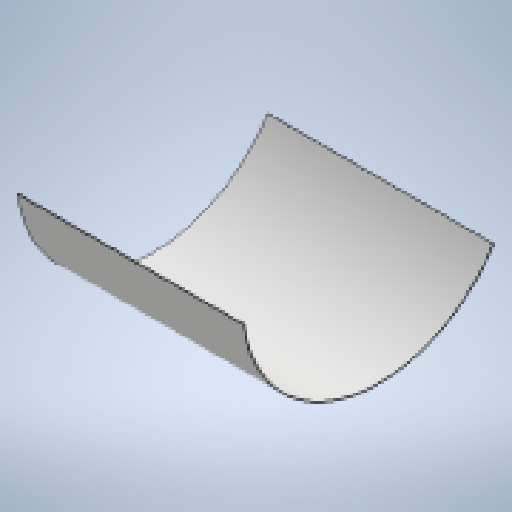
# Autodesk Inventor part: TRM 027 tromel
Saved by Autodesk Inventor 2025 (Build 290162010, 162A)
## iProperties
Created: 2024-08-07
Part Number: TRM 027 tromel
Material: AISI 304
Document SubType Name: Sheet Metal
Designer: admin
Stock Number: ТРМ 017 лист внутри
Density: 8.02768 g/cm^3
Flat Pattern Width: 50 cm
Flat Pattern Length: 73.7116 cm
Flat Pattern Area: 3685.58 cm^2
Sheet Metal Rule: AISI304 2mm Die16
Sheet Metal Width: 500,000 mm
Sheet Metal Length: 737,116 mm
Sheet Metal Area: 368558,013 mm^2
Appearance: Default
d73_joint_angle: 7,40 deg
Author: pokla
Autodesk Inventor part; units mm, degrees
ref_plane "YZ Plane" through (0, 0, 0) normal (1, 0, 0) x (0, 1, 0)
ref_plane "XZ Plane" through (0, 0, 0) normal (0, 1, 0) x (-1, 0, 0)
ref_plane "XY Plane" through (0, 0, 0) normal (0, 0, 1) x (1, 0, 0)
sketch "Sketch7" plane through (0, 0, 0) normal (1, 0, 0) x (0, 1, 0)
  line L0 (297.5, 0) -> (-297.5, 0) construction
  arc A0 (-297.5, 0) -> (253.7716, -121.3509) centre (0, 38.6491) ccw
  line L1 (-253.7716, -121.3509) -> (253.7716, -121.3509) construction
  arc A1 (253.7716, -121.3509) -> (297.5, 0) centre (0, 38.6491) ccw construction
  line L2 (-297.5, 0) -> (-263.5472, -261.3509) construction
  line L3 (-297.5, 0) -> (-297.5, -261.3509) construction
  line L4 (-297.5, -261.3509) -> (165.5032, -261.3509) construction
  line L5 (253.7716, -121.3509) -> (165.5032, -261.3509) construction
  line L6 (-297.5, 0) -> (-310.383, 99.1667)
  line L7 (253.7716, -121.3509) -> (253.7716, 0) construction
  point P0 (0, 0)
  point P1 (0, 0)
  point P2 (-123.3439, -261.3509)
  dimension "d54" = 300
  dimension "d66" = 121.3509
  dimension "d68" = 7.402
  dimension "d69" = 595
  dimension "d70" = 140
  dimension "d72" = 100
  dimension "d73_joint_angle" = 7.402
  dimension "d74" = 147.769
  measures "d54" radius of A0
  measures "d66" distance between parallel lines of L1 L0
  measures "d68" angle of L2 L3
  measures "d69" distance of L0.start L0.end
  measures "d70" distance from line of point (-123.344, -261.351) L1
  measures "d72" distance of L0.end L6.end
  measures "d73_joint_angle" angle of L6 L3
  measures "d74" angle of L7 L5
contour flange "Contour Flange1" sketch "Sketch7" thickness 2 bend radius 2.75 width 500 along (1, 0, 0) mid plane no both sides no wall seen from (0, -64.4946, -254.3363) lies toward (0, -0.2149821, -0.976618) curves A0
bend "Bend5"
corner "Corner5"
equation "\"d55\" = Thickness"
equation "\"d56\" = BendReliefWidth"
equation "\"d57\" = BendReliefDepth"
equation "\"d58\" = MinimumRemnant"
equation "\"d59\" = TransitionRadius"
equation "\"d61\" = BendRadius"
equation "\"d63\" = CornerReliefSize"
equation "\"d64\" = GapSize"
equation "\"d65\" = JacobiRadiusSize"
equation "\"BendReliefWidth\" = Thickness"
equation "\"BendReliefDepth\" = 0.5 * Thickness"
equation "\"CornerReliefSize\" = 4 * Thickness"
equation "\"MinimumRemnant\" = 2 * Thickness"
equation "\"TransitionRadius\" = BendRadius"
equation "\"JacobiRadiusSize\" = BendRadius"
equation "\"GapSize\" = Thickness"
equation "\"Thickness\" = 2"
equation "\"BendRadius\" = 2.75"
body "Solid2"
